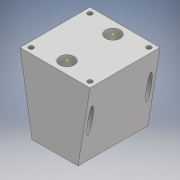
# Autodesk Inventor part: RDtoRC2-height40mm
Saved by Autodesk Inventor 2017 (Build 210142000, 142)
## iProperties
Created: 2021-10-11
Part Number: RDtoRC2-height40mm
Material: Generic
Document SubType Name: Modeling
Designer: Nikita
Density: 1 g/cm^3
Appearance: Default
Author: Nikita
Autodesk Inventor part; units mm, degrees
ref_plane "YZ Plane" through (0, 0, 0) normal (1, 0, 0) x (0, 1, 0)
ref_plane "XZ Plane" through (0, 0, 0) normal (0, 1, 0) x (-1, 0, 0)
ref_plane "XY Plane" through (0, 0, 0) normal (0, 0, 1) x (1, 0, 0)
sketch "Sketch1" plane through (0, 0, 0) normal (0, 0, 1) x (1, 0, 0)
  line L0 (12.5, -19) -> (-12.5, -19)
  line L1 (-12.5, -19) -> (-12.5, 19)
  line L2 (-12.5, 19) -> (12.5, 19)
  line L3 (12.5, 19) -> (12.5, -19)
  line L4 (12.5, -19) -> (-12.5, 19) construction
  line L5 (-12.5, -19) -> (12.5, 19) construction
  circle A0 centre (0, 12.5) radius 2.1
  circle A1 centre (0, -12.5) radius 2.1
  point P0 (0, 0)
  dimension "d0" = 25
  dimension "d1" = 38
  dimension "d2" = 4.2
  dimension "d3" = 4.2
  dimension "d4" = 12.5
  dimension "d5" = 12.5
  constraints: 12 end point, 2 centre point, 2 midpoint, 2 parallel, 1 horizontal, 1 perpendicular
  measures "d0" distance of L1.end L2.end
  measures "d1" distance of L0.end L1.end
  measures "d2" diameter of A0
  measures "d3" diameter of A1
  measures "d4" distance of point (0, 0) A0.centre
  measures "d5" distance of A1.centre point (0, 0)
extrude "Extrusion1" add sketch "Sketch1" along normal blind 40
sketch "Sketch2" plane through (-12.5, 19, 0) normal (0, 1, 0) x (1, 0, 0)
  line L0 (0, 0) -> (0, -40) projected
  line L1 (0, -40) -> (-6.5, -40)
  line L2 (-6.5, -40) -> (0, 0)
  line L3 (0, -40) -> (25, -40) projected
  line L4 (0, 0) -> (0, -40)
  line L5 (25, -40) -> (31.5, -40)
  line L6 (25, 0) -> (25, -40) projected
  line L7 (31.5, -40) -> (25, 0)
  line L8 (25, 0) -> (25, -40)
  point P0 (12.5, 0)
  dimension "d8" = 6.5
  dimension "d9" = 6.5
  constraints: 12 end point, 2 horizontal, 2 perpendicular
  measures "d8" distance of L0.end L1.end
  measures "d9" distance of L3.end L5.end
extrude "Extrusion2" add sketch "Sketch2" against normal up to surface (38 mm away)
sketch "Sketch3" plane through (0, 0, 40) normal (0, 0, 1) x (1, 0, 0)
  line L0 (-5.4088, 0) -> (7.7062, 0)
  line L1 (0, 5.8117) -> (0, -6.6687)
  point P0 (0, 0)
  point P1 (-16, 16)
  point P2 (16, 16)
  point P3 (-16, -16)
  point P4 (16, -16)
  dimension "d12" = 16
  dimension "d13" = 16
  dimension "d16" = 32
  dimension "d19" = 32
  constraints: 4 end point, 2 horizontal, 1 perpendicular, 1 vertical, 3 other
  measures "d12" horizontal distance of point (0, 0) point (-16, 16)
  measures "d13" horizontal distance of point (0, 0) point (-16, 16)
  measures "d16" distance of point (-16, 16) point (16, 16)
  measures "d19" distance of point (-16, 16) point (-16, -16)
hole "Hole1" at (-16, 16, 40) at (16, 16, 40) at (-16, -16, 40) at (16, -16, 40) direction (0, 0, -1) diameter 2.5 end through all
hole "Hole2" at (0, -12.5, 40) direction (0, 0, -1) diameter 8 depth 36 tip angle 118
hole "Hole3" at (0, 12.5, 40) direction (0, 0, -1) diameter 8 depth 36 tip angle 118
body "Solid1"
